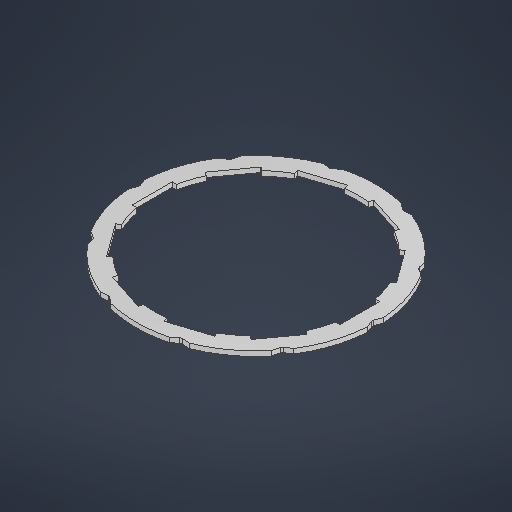
# Autodesk Inventor part: lamina_rotor
Saved by Autodesk Inventor 2025 (Build 290162010, 162A)
## iProperties
Created: 2024-11-09
Part Number: lamina_rotor
Material: Generic
Document SubType Name: Modeling
Designer: river
Density: 1 g/cm^3
Appearance: Default
Finish1_Area: 11622,603 mm^2
Finish1_Appearance: Aluminum - Dark
Author: river
Autodesk Inventor part; units mm, degrees
ref_plane "YZ Plane" through (0, 0, 0) normal (1, 0, 0) x (0, 1, 0)
ref_plane "XZ Plane" through (0, 0, 0) normal (0, 1, 0) x (-1, 0, 0)
ref_plane "XY Plane" through (0, 0, 0) normal (0, 0, 1) x (1, 0, 0)
sketch "Sketch1" plane through (0, 0, 0) normal (0, 1, 0) x (-1, 0, 0)
  circle A0 centre (0, 0) radius 75
  circle A1 centre (0, 0) radius 63.5
  line L0 (62, 12.5) -> (62, -12.5)
  line L1 (62, -12.5) -> (65, -12.5)
  line L2 (65, -12.5) -> (65, 12.5)
  line L3 (65, 12.5) -> (62, 12.5)
  line L4 (62, 12.5) -> (65, -12.5) construction
  line L5 (62, -12.5) -> (65, 12.5) construction
  line L6 (75, 0) -> (0, 0) construction
  line L7 (59.9334, 28.0933) -> (45.2388, 48.3188)
  line L8 (45.2388, 48.3188) -> (42.8117, 46.5554)
  line L9 (42.8117, 46.5554) -> (57.5064, 26.33)
  line L10 (57.5064, 26.33) -> (59.9334, 28.0933)
  line L11 (31.9743, 57.956) -> (8.1979, 65.6814)
  line L12 (8.1979, 65.6814) -> (7.2708, 62.8282)
  line L13 (7.2708, 62.8282) -> (31.0473, 55.1028)
  line L14 (31.0473, 55.1028) -> (31.9743, 57.956)
  line L15 (-8.1979, 65.6814) -> (-31.9743, 57.956)
  line L16 (-31.9743, 57.956) -> (-31.0473, 55.1028)
  line L17 (-31.0473, 55.1028) -> (-7.2708, 62.8282)
  line L18 (-7.2708, 62.8282) -> (-8.1979, 65.6814)
  line L19 (-45.2388, 48.3188) -> (-59.9334, 28.0933)
  line L20 (-59.9334, 28.0933) -> (-57.5064, 26.33)
  line L21 (-57.5064, 26.33) -> (-42.8117, 46.5554)
  line L22 (-42.8117, 46.5554) -> (-45.2388, 48.3188)
  line L23 (-65, 12.5) -> (-65, -12.5)
  line L24 (-65, -12.5) -> (-62, -12.5)
  line L25 (-62, -12.5) -> (-62, 12.5)
  line L26 (-62, 12.5) -> (-65, 12.5)
  line L27 (-59.9334, -28.0933) -> (-45.2388, -48.3188)
  line L28 (-45.2388, -48.3188) -> (-42.8117, -46.5554)
  line L29 (-42.8117, -46.5554) -> (-57.5064, -26.33)
  line L30 (-57.5064, -26.33) -> (-59.9334, -28.0933)
  line L31 (-31.9743, -57.956) -> (-8.1979, -65.6814)
  line L32 (-8.1979, -65.6814) -> (-7.2708, -62.8282)
  line L33 (-7.2708, -62.8282) -> (-31.0473, -55.1028)
  line L34 (-31.0473, -55.1028) -> (-31.9743, -57.956)
  line L35 (8.1979, -65.6814) -> (31.9743, -57.956)
  line L36 (31.9743, -57.956) -> (31.0473, -55.1028)
  line L37 (31.0473, -55.1028) -> (7.2708, -62.8282)
  line L38 (7.2708, -62.8282) -> (8.1979, -65.6814)
  line L39 (45.2388, -48.3188) -> (59.9334, -28.0933)
  line L40 (59.9334, -28.0933) -> (57.5064, -26.33)
  line L41 (57.5064, -26.33) -> (42.8117, -46.5554)
  line L42 (42.8117, -46.5554) -> (45.2388, -48.3188)
  circle A2 centre (75, 0) radius 2
  line L43 (74.8331, 5) -> (73.1411, 0.738)
  line L44 (73.1411, -0.738) -> (74.8331, -5)
  circle A3 centre (60.6763, 44.0839) radius 2
  line L45 (57.6024, 48.0309) -> (58.7386, 43.5883)
  line L46 (59.6062, 42.3942) -> (63.4802, 39.9407)
  circle A4 centre (23.1763, 71.3292) radius 2
  line L47 (18.3694, 72.7156) -> (21.9, 69.7894)
  line L48 (23.3037, 69.3333) -> (27.88, 69.6255)
  circle A5 centre (-23.1763, 71.3292) radius 2
  line L49 (-27.88, 69.6255) -> (-23.3037, 69.3333)
  line L50 (-21.9, 69.7894) -> (-18.3694, 72.7156)
  circle A6 centre (-60.6763, 44.0839) radius 2
  line L51 (-63.4802, 39.9407) -> (-59.6062, 42.3942)
  line L52 (-58.7386, 43.5883) -> (-57.6024, 48.0309)
  circle A7 centre (-75, 0) radius 2
  line L53 (-74.8331, -5) -> (-73.1411, -0.738)
  line L54 (-73.1411, 0.738) -> (-74.8331, 5)
  circle A8 centre (-60.6763, -44.0839) radius 2
  line L55 (-57.6024, -48.0309) -> (-58.7386, -43.5883)
  line L56 (-59.6062, -42.3942) -> (-63.4802, -39.9407)
  circle A9 centre (-23.1763, -71.3292) radius 2
  line L57 (-18.3694, -72.7156) -> (-21.9, -69.7894)
  line L58 (-23.3037, -69.3333) -> (-27.88, -69.6255)
  circle A10 centre (23.1763, -71.3292) radius 2
  line L59 (27.88, -69.6255) -> (23.3037, -69.3333)
  line L60 (21.9, -69.7894) -> (18.3694, -72.7156)
  circle A11 centre (60.6763, -44.0839) radius 2
  line L61 (63.4802, -39.9407) -> (59.6062, -42.3942)
  line L62 (58.7386, -43.5883) -> (57.6024, -48.0309)
  point P0 (63.5, 0)
  point P1 (63.5, 0)
  point P2 (62.2575, -12.5)
  point P3 (57.7147, -26.4813)
  point P4 (43.0201, -46.7068)
  point P5 (31.1268, -55.3477)
  point P6 (7.3504, -63.0731)
  point P7 (-7.3504, -63.0731)
  point P8 (-31.1268, -55.3477)
  point P9 (-43.0201, -46.7068)
  point P10 (-57.7147, -26.4813)
  point P11 (-62.2575, -12.5)
  point P12 (-62.2575, 12.5)
  point P13 (-57.7147, 26.4813)
  point P14 (-43.0201, 46.7068)
  point P15 (-31.1268, 55.3477)
  point P16 (-7.3504, 63.0731)
  point P17 (7.3504, 63.0731)
  point P18 (31.1268, 55.3477)
  point P19 (43.0201, 46.7068)
  point P20 (57.7147, 26.4813)
  point P21 (62.2575, 12.5)
  point P22 (65, 0)
  dimension "d1" = 127
  dimension "d2" = 25
  dimension "d3" = 3
  dimension "d6" = 360
  dimension "d11" = 4
  dimension "d12" = 10
  dimension "d13" = 5
  dimension "d15" = 10
  dimension "d16" = 150
  dimension "d19" = 360
  constraints: 126 end point, 23 point on circle, 11 centre point, 3 coincident, 3 midpoint, 2 parallel, 2 tangent, 1 horizontal, 1 perpendicular, 1 point on line, 1 vertical, 165 other
  measures "d2" distance of L0.start L0.end
  measures "d3" distance of L1.end L0.end
  measures "d11" diameter of A2
  measures "d12" distance of L44.end L43.start
  measures "d13" vertical distance of L43.start L6.start
  measures "d15" distance of point (65, 0) L6.start
  measures "d16" diameter of A0
extrude "Extrusion1" add sketch "Sketch1" along normal blind 3 contours L43 A2 L44 A0 L61 A11 L62 L59 A10 L60 L57 A9 L58 L55 A8 L56 L53 A7 L54 L51 A6 L52 L49 A5 L50 L47 A4 L48 L45 A3 L46
body "Solid1"
